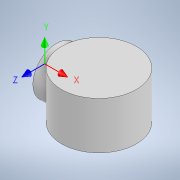
# Autodesk Inventor part: hip
Saved by Autodesk Inventor 2020.2 (Build 242310000, 310)
## iProperties
Created: 2021-01-29
Part Number: hip
Material: Generic
Document SubType Name: Modeling
Designer: DELL
Density: 1 g/cm^3
Appearance: Default
Author: DELL
Autodesk Inventor part; units mm, degrees
ref_plane "YZ Plane" through (0, 0, 0) normal (1, 0, 0) x (0, 1, 0)
ref_plane "XZ Plane" through (0, 0, 0) normal (0, 1, 0) x (-1, 0, 0)
ref_plane "XY Plane" through (0, 0, 0) normal (0, 0, 1) x (1, 0, 0)
sketch "Sketch1" plane through (0, 0, 0) normal (1, 0, 0) x (0, 1, 0)
  circle A0 centre (0, 0) radius 30
  dimension "d0" = 60
  constraints: 1 centre point, 1 coincident
  measures "d0" diameter of A0
extrude "Extrusion1" add sketch "Sketch1" along normal blind 54
sketch "Sketch2" plane through (0, 0, 0) normal (0, 1, 0) x (-1, 0, 0)
  line L0 (-54, 30) -> (-54, -30) projected
  circle A0 centre (-54, 0) radius 47.5
  point P0 (0, 0)
  dimension "d3" = 95
  constraints: 1 centre point, 1 midpoint
  measures "d3" diameter of A0
extrude "Extrusion2" add sketch "Sketch2" along normal mid plane 60
move or copy body "Move Body1" bodies to move or copy 1 copy no translate (15, 0, 0)
body "Solid1"
